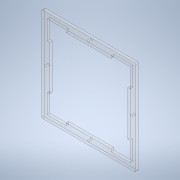
# Autodesk Inventor part: WaagePlexiMittelsteuck
Saved by Autodesk Inventor 2022 (Build 260153000, 153)
## iProperties
Created: 2021-12-03
Part Number: WaagePlexiMittelsteuck
Material: PET Plastic
Document SubType Name: Modeling
Designer: domin
Density: 1.541 g/cm^3
Appearance: Polycarbonate - Clear
Mass: 65.5796 g
Surface Area: 241.368 cm^2
Volume: 42.5565 cm^3
Author: domin
Autodesk Inventor part; units mm, degrees
ref_plane "YZ Plane" through (0, 0, 0) normal (1, 0, 0) x (0, 1, 0)
ref_plane "XZ Plane" through (0, 0, 0) normal (0, 1, 0) x (-1, 0, 0)
ref_plane "XY Plane" through (0, 0, 0) normal (0, 0, 1) x (1, 0, 0)
sketch "Sketch1" plane through (0, 0, 0) normal (0, 0, 1) x (1, 0, 0)
  line L0 (-89, 89) -> (89, 89)
  line L1 (89, 89) -> (89, -89)
  line L2 (89, -89) -> (-89, -89)
  line L3 (-89, -89) -> (-89, 89)
  line L4 (-78.5, 42.5) -> (-74, 42.5)
  line L5 (-74, 42.5) -> (-74, -42.5)
  line L6 (-74, -42.5) -> (-78.5, -42.5)
  line L7 (42.5, 78.5) -> (42.5, 74)
  line L8 (42.5, 74) -> (-42.5, 74)
  line L9 (-42.5, 74) -> (-42.5, 78.5)
  line L10 (78.5, 42.5) -> (74, 42.5)
  line L11 (74, 42.5) -> (74, -42.5)
  line L12 (74, -42.5) -> (78.5, -42.5)
  line L13 (42.5, -78.5) -> (42.5, -74)
  line L14 (42.5, -74) -> (-42.5, -74)
  line L15 (-42.5, -74) -> (-42.5, -78.5)
  line L16 (-78.5, 78.5) -> (-42.5, 78.5)
  line L17 (42.5, 78.5) -> (78.5, 78.5)
  line L18 (-78.5, -78.5) -> (-78.5, -42.5)
  line L19 (-78.5, 42.5) -> (-78.5, 78.5)
  line L20 (78.5, -78.5) -> (42.5, -78.5)
  line L21 (-42.5, -78.5) -> (-78.5, -78.5)
  line L22 (78.5, 78.5) -> (78.5, 42.5)
  line L23 (78.5, -42.5) -> (78.5, -78.5)
  point P0 (0, 0)
  point P1 (-74, 0)
  point P2 (0, 74)
  dimension "d0" = 36
  dimension "d1" = 36
  dimension "d2" = 148
  dimension "d3" = 148
  dimension "d4" = 157
  dimension "d5" = 157
  dimension "d6" = 74
  dimension "d7" = 74
  dimension "d9" = 15
  dimension "d14" = 15
  dimension "d15" = 15
  constraints: 48 end point, 14 parallel, 7 perpendicular, 6 horizontal, 5 horizontal alignment, 5 vertical alignment, 3 equal length, 2 midpoint, 2 point on line
  measures "d0" distance between parallel lines of L9 L19
  measures "d1" distance between parallel lines of L4 L16
  measures "d2" distance between parallel lines of L11 L5
  measures "d3" distance between parallel lines of L14 L8
  measures "d4" distance between parallel lines of L21 L16
  measures "d5" distance between parallel lines of L19 L22
  measures "d6" distance from line of point (0, 0) L8
  measures "d7" distance from line of point (0, 0) L5
  measures "d9" distance between parallel lines of L3 L5
  measures "d14" distance between parallel lines of L0 L8
  measures "d15" distance between parallel lines of L1 L11
extrude "Extrusion1" add sketch "Sketch1" along normal blind 5
sketch "Sketch2" plane through (0, 0, 5) normal (0, 0, 1) x (1, 0, 0)
  circle A0 centre (-81.5, 0) radius 2
  circle A1 centre (81.5, 0) radius 2
  line L0 (-74, -42.5) -> (-74, 42.5) projected
  line L1 (74, 42.5) -> (74, -42.5) projected
  circle A2 centre (0, 81.5) radius 2
  circle A3 centre (0, -81.5) radius 2
  line L2 (-42.5, 74) -> (42.5, 74) projected
  line L3 (42.5, -74) -> (-42.5, -74) projected
  point P0 (0, 0)
  dimension "d16" = 7.5
  dimension "d17" = 7.5
  dimension "d18" = 4
  dimension "d19" = 7.5
  dimension "d20" = 7.5
  constraints: 4 centre point, 3 equal radius, 2 horizontal alignment, 2 vertical alignment
  measures "d16" distance from line of A0.centre L0
  measures "d17" distance from line of L1 A1.centre
  measures "d18" diameter of A0
  measures "d19" distance from line of L2 A2.centre
  measures "d20" distance from line of L3 A3.centre
hole "Hole1" at (-81.5, 0, 5) at (0, 81.5, 5) at (81.5, 0, 5) at (0, -81.5, 5) direction (0, 0, -1) diameter 4 end through all
fillet "Fillet1" radius 2 4 edges at (-89, -89, 2.5) (-89, 89, 2.5) (89, -89, 2.5) (89, 89, 2.5)
equation "\"d6\" = 0.5 * d3"
equation "\"d7\" = 0.5 * d2"
equation "\"d21\" = d18"
body "Solid1"
